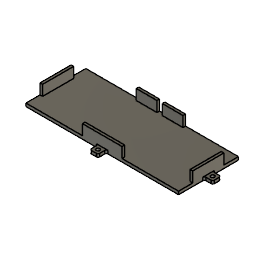
SNES Cradle (Autodesk Fusion 360 design; units mm, degrees)
part number: 2026-08-31-20-38-05-877
Autodesk Fusion 360 part; units mm, degrees
sketch "Sketch2" plane through (0, 0, 0) normal (0, 0, 1) x (1, 0, 0)
  line L0 (0, 0) -> (146.5, 0)
  line L1 (146.5, 0) -> (146.5, 57.5)
  line L2 (146.5, 57.5) -> (0, 57.5)
  line L3 (0, 57.5) -> (0, 0)
  line L4 (69.25, 0) -> (77.25, 0)
  line L5 (77.25, 0) -> (77.25, -8)
  line L6 (77.25, -8) -> (69.25, -8)
  line L7 (69.25, -8) -> (69.25, 0)
  line L8 (146.5, 24.75) -> (146.5, 32.75)
  line L9 (146.5, 32.75) -> (154.5, 32.75)
  line L10 (154.5, 32.75) -> (154.5, 24.75)
  line L11 (154.5, 24.75) -> (146.5, 24.75)
  line L12 (73.25, 57.5) -> (73.25, 0) construction
  line L13 (146.5, 28.75) -> (154.5, 28.75) construction
  line L14 (150.5, 32.75) -> (150.5, 24.75) construction
  circle A0 centre (150.5, 28.75) radius 1.75
  line L15 (-8, 24.75) -> (0, 24.75)
  line L16 (-8, 32.75) -> (-8, 24.75)
  line L17 (0, 32.75) -> (-8, 32.75)
  circle A1 centre (-4, 28.75) radius 1.75
  line L18 (69.25, -4) -> (77.25, -4) construction
  line L19 (73.25, 0) -> (73.25, -8) construction
  circle A2 centre (73.25, -4) radius 1.75
  point P0 (73.25, 0)
  point P1 (146.5, 28.75)
  point P2 (-8, 28.75)
  dimension "d8" = 146.5
  dimension "d9" = 57.5
  dimension "d12" = 8
  dimension "d13" = 8
  dimension "d14" = 8
  dimension "d15" = 8
  dimension "d16" = 8
  dimension "d17" = 3.5
  dimension "d18" = 3.5
  constraint horizontal L0
  constraint vertical L1
  constraint horizontal L2
  constraint vertical L3
  constraint coincident L0.start L3.end
  constraint midpoint L4 P0
  constraint coincident L0 P0
  constraint coincident L0 L4.end
  constraint perpendicular L4 L5
  constraint perpendicular L5 L6
  constraint midpoint L8 P1
  constraint coincident L1 P1
  constraint parallel L1 L8
  constraint perpendicular L1 L9
  constraint perpendicular L9 L10
  constraint midpoint L2 L12.start
  constraint coincident P0 L12.end
  constraint perpendicular L0 L12
  constraint coincident P1 L13.start
  constraint midpoint L10 L13.end
  constraint midpoint L9 L14.start
  constraint midpoint L11 L14.end
  constraint midpoint L13 A0.centre
  constraint symmetric L8.start L12 L15.end
  constraint symmetric L8.end L12 L17.start
  constraint symmetric L9.end L12 L16.start
  constraint symmetric L10.end L12 L15.start
  constraint symmetric L12 L13.end P2
  constraint symmetric L12 A0 A1
  constraint midpoint L7 L18.start
  constraint midpoint L5 L18.end
  constraint midpoint L6 L19.end
  constraint midpoint L19 A2.centre
  measures "d8" distance of L0.start L0.end
  measures "d9" distance of L0.start L2.end
  measures "d12" distance of L4.start L4.end
  measures "d13" distance of L5.end L6.end
  measures "d14" distance of L8.start L8.end
  measures "d15" distance of L8.end L9.end
  measures "d16" distance of L9.end L10.end
  measures "d17" diameter of A0
  measures "d18" diameter of A2
extrude "Extrude1" add sketch "Sketch2" along normal blind 3
fillet "Fillet1" radius 1.5 12 edges at (77.25, 0, 1.5) (77.25, -8, 1.5) (69.25, -8, 1.5) (69.25, 0, 1.5) (0, 24.75, 1.5) (-8, 24.75, 1.5) (-8, 32.75, 1.5) (0, 32.75, 1.5) (154.5, 32.75, 1.5) (146.5, 32.75, 1.5) (146.5, 24.75, 1.5) (154.5, 24.75, 1.5)
sketch "Sketch3" plane through (0, 0, 3) normal (0, 0, 1) x (-1, 0, 0)
  arc A0 (-153, -24.75) -> (-154.5, -26.25) centre (-153, -26.25) ccw
  line L0 (-154.5, -26.25) -> (-154.5, -31.25)
  arc A1 (-154.5, -31.25) -> (-153, -32.75) centre (-153, -31.25) ccw
  line L1 (-153, -32.75) -> (-148, -32.75)
  arc A2 (-146.5, -34.25) -> (-148, -32.75) centre (-148, -34.25) ccw
  line L2 (-146.5, -34.25) -> (-146.5, -57.5)
  line L3 (-146.5, -57.5) -> (0, -57.5)
  line L4 (0, -57.5) -> (0, -34.25)
  arc A3 (1.5, -32.75) -> (0, -34.25) centre (1.5, -34.25) ccw
  line L5 (1.5, -32.75) -> (6.5, -32.75)
  arc A4 (6.5, -32.75) -> (8, -31.25) centre (6.5, -31.25) ccw
  line L6 (8, -31.25) -> (8, -26.25)
  arc A5 (8, -26.25) -> (6.5, -24.75) centre (6.5, -26.25) ccw
  line L7 (6.5, -24.75) -> (1.5, -24.75)
  arc A6 (0, -23.25) -> (1.5, -24.75) centre (1.5, -23.25) ccw
  line L8 (0, -23.25) -> (0, 0)
  line L9 (0, 0) -> (-67.75, 0)
  arc A7 (-69.25, 1.5) -> (-67.75, 0) centre (-67.75, 1.5) ccw
  line L10 (-69.25, 1.5) -> (-69.25, 6.5)
  arc A8 (-69.25, 6.5) -> (-70.75, 8) centre (-70.75, 6.5) ccw
  line L11 (-70.75, 8) -> (-75.75, 8)
  arc A9 (-75.75, 8) -> (-77.25, 6.5) centre (-75.75, 6.5) ccw
  line L12 (-77.25, 6.5) -> (-77.25, 1.5)
  arc A10 (-78.75, 0) -> (-77.25, 1.5) centre (-78.75, 1.5) ccw
  line L13 (-78.75, 0) -> (-146.5, 0)
  line L14 (-146.5, 0) -> (-146.5, -23.25)
  arc A11 (-148, -24.75) -> (-146.5, -23.25) centre (-148, -23.25) ccw
  line L15 (-148, -24.75) -> (-153, -24.75)
  circle A12 centre (-150.5, -28.75) radius 1.75
  circle A13 centre (4, -28.75) radius 1.75
  circle A14 centre (-73.25, 4) radius 1.75
  line L16 (0, -2.5) -> (-146.5, -2.5) construction
  line L17 (-54.25, -2.5) -> (-92.25, -2.5)
  line L18 (-92.25, -2.5) -> (-92.25, 0)
  line L19 (-54.25, -2.5) -> (-54.25, 0)
  line L20 (-54.25, 0) -> (-92.25, 0)
  line L21 (-144, -57) -> (-144, 0) construction
  line L22 (-144, -13.5) -> (-144, -43.5)
  line L23 (-144, -43.5) -> (-146.5, -43.5)
  line L24 (-144, -13.5) -> (-146.5, -13.5)
  line L25 (-146.5, -13.5) -> (-146.5, -43.5)
  line L26 (-73.25, -57.5) -> (-73.25, 0) construction
  line L27 (-2.5, -13.5) -> (0, -13.5)
  line L28 (0, -13.5) -> (0, -43.5)
  line L29 (-2.5, -43.5) -> (0, -43.5)
  line L30 (-2.5, -13.5) -> (-2.5, -43.5)
  line L31 (0, -55) -> (-146.5, -55) construction
  line L32 (-50.75, -55) -> (-95.75, -55)
  line L33 (-95.75, -55) -> (-95.75, -57.5)
  line L34 (-50.75, -55) -> (-50.75, -57.5)
  line L35 (-50.75, -57.5) -> (-95.75, -57.5)
  line L36 (-70.75, -55) -> (-75.75, -55)
  line L37 (-75.75, -55) -> (-75.75, -57.5)
  line L38 (-75.75, -57.5) -> (-70.75, -57.5)
  line L39 (-70.75, -57.5) -> (-70.75, -55)
  point P0 (-73.25, -2.5)
  point P1 (-144, -28.5)
  point P2 (-73.25, -55)
  point P3 (-73.25, -55)
  dimension "d23" = 2.5
  dimension "d24" = 38
  dimension "d25" = 2.5
  dimension "d26" = 30
  dimension "d27" = 2.5
  dimension "d28" = 45
  dimension "d29" = 5
  constraint coincident L8 L16.start
  constraint coincident L14 L16.end
  constraint perpendicular L14 L16
  constraint midpoint L17 P0
  constraint coincident L16 P0
  constraint parallel L16 L17
  constraint coincident L13 L18.end
  constraint perpendicular L13 L18
  constraint coincident L9 L19.end
  constraint perpendicular L9 L19
  constraint coincident L13 L21.end
  constraint perpendicular L13 L21
  constraint midpoint L22 P1
  constraint coincident L21 P1
  constraint perpendicular L15 L22
  constraint coincident L2 L23.end
  constraint perpendicular L2 L23
  constraint coincident L14 L24.end
  constraint perpendicular L14 L24
  constraint midpoint L3 L26.start
  constraint midpoint L20 L26.end
  constraint symmetric L22.start L26 L27.start
  constraint symmetric L22.end L26 L29.start
  constraint symmetric L23.end L26 L28.end
  constraint symmetric L24.end L26 L27.end
  constraint coincident L4 L31.start
  constraint coincident L2 L31.end
  constraint perpendicular L2 L31
  constraint midpoint L32 P3
  constraint coincident L31 P3
  constraint perpendicular L26 L32
  constraint coincident L3 L33.end
  constraint perpendicular L3 L33
  constraint coincident L3 L34.end
  constraint perpendicular L3 L34
  constraint midpoint L36 P3
  constraint coincident P3 P2
  constraint perpendicular L26 L36
  constraint coincident L35 L37.end
  constraint coincident L35 L38.end
  measures "d23" distance of L9 L16
  measures "d24" distance of L17.start L17.end
  measures "d25" distance of L14 L21
  measures "d26" distance of L22.start L22.end
  measures "d27" distance of L3 L31
  measures "d28" distance of L32.start L32.end
  measures "d29" distance of L36.start L36.end
extrude "Extrude2" add sketch "Sketch3" along normal blind 10 contours L2 L14 L22 L23 L24 L25 | L9 L13 L17 L18 L19 L20 | L3 L32 L33 L35 L37 | L3 L32 L34 L35 L39 | L4 L8 L27 L28 L29 L30
equation "controller_length = 143 mm"
equation "controller_width = 54 mm"
equation "mount_hole_diameter = 3.5 mm"
equation "base_thickness = 3 mm"
equation "wall_thickness = 2.5 mm"
equation "give = 1 mm"
equation "d8 = total_length"
equation "d9 = total_width"
equation "total_length = controller_length + wall_thickness + give"
equation "total_width = controller_width + give + wall_thickness"
equation "d19 = base_thickness"
equation "d23 = wall_thickness"
equation "d25 = wall_thickness"
equation "d27 = wall_thickness"
